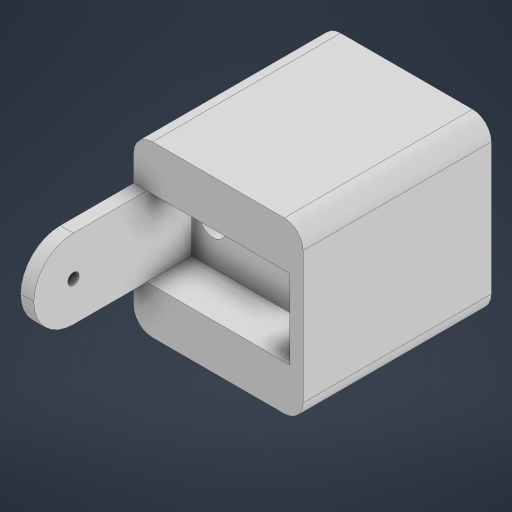
# Autodesk Inventor part: Motor holder
Saved by Autodesk Inventor 2023 (Build 270158000, 158)
## iProperties
Created: 2023-04-10
Part Number: Motor holder
Material: Generic
Document SubType Name: Modeling
Designer: vatdu
Density: 1 g/cm^3
Appearance: Default
Author: vatdu
Autodesk Inventor part; units mm, degrees
ref_plane "YZ Plane" through (0, 0, 0) normal (1, 0, 0) x (0, 1, 0)
ref_plane "XZ Plane" through (0, 0, 0) normal (0, 1, 0) x (-1, 0, 0)
ref_plane "XY Plane" through (0, 0, 0) normal (0, 0, 1) x (1, 0, 0)
sketch "Sketch1" plane through (0, 0, 0) normal (0, 0, 1) x (1, 0, 0)
  line L0 (0, 0) -> (45, 0)
  line L1 (45, 0) -> (45, 45)
  line L2 (45, 45) -> (0, 45)
  line L3 (0, 45) -> (0, 0)
  dimension "d0" = 45
  dimension "d1" = 45
  constraints: 8 end point, 2 parallel, 1 horizontal, 1 perpendicular
  measures "d0" distance of L2.end L1.end
  measures "d1" distance of L1.end L0.end
extrude "Extrusion1" add sketch "Sketch1" along normal blind 50
fillet "Fillet1" radius 5 4 edges at (45, 45, 25) (0, 45, 25) (45, 0, 25) (0, 0, 25)
sketch "Sketch2" plane through (0, 0, 0) normal (0, 0, -1) x (-1, 0, 0)
  line L0 (-45, 5) -> (-45, 40) projected
  line L1 (-45, 22.5) -> (-22.5, 22.5)
  circle A0 centre (-22.5, 22.5) radius 7.5
  point P0 (0, 0)
  dimension "d5" = 22.5
  dimension "d6" = 15
  constraints: 2 end point, 1 centre point, 1 coincident, 1 horizontal, 1 midpoint
  measures "d5" distance of L1.start L1.end
  measures "d6" diameter of A0
extrude "Extrusion2" cut sketch "Sketch2" against normal blind 20
sketch "Sketch3" plane through (0, 0, 50) normal (0, 0, 1) x (1, 0, 0)
  line L0 (0, 0) -> (3.5, 0)
  line L1 (5, 0) -> (40, 0) projected
  line L2 (3.5, 0) -> (3.5, 12)
  line L3 (3.5, 12) -> (41.5, 12)
  line L4 (41.5, 12) -> (41.5, 33)
  line L5 (41.5, 33) -> (3.5, 33)
  line L6 (3.5, 33) -> (3.5, 12)
  dimension "d11" = 3.5
  dimension "d12" = 12
  dimension "d13" = 38
  dimension "d14" = 21
  constraints: 12 end point, 2 parallel, 2 perpendicular, 1 collinear, 1 horizontal
  measures "d11" distance of L0.start L0.end
  measures "d12" distance of L0.end L2.end
  measures "d13" distance of L5.end L4.end
  measures "d14" distance of L4.end L3.end
extrude "Extrusion3" cut sketch "Sketch3" against normal blind 12
sketch "Sketch4" plane through (0, 0, 38) normal (0, 0, 1) x (1, 0, 0)
  line L0 (3.5, 12) -> (3.5, 33) projected
  line L1 (3.5, 22.5) -> (29.5, 22.5)
  line L2 (29.5, 22.5) -> (33.5, 22.5)
  line L3 (3.5, 33) -> (41.5, 33) projected
  line L4 (30.5, 33) -> (37.7775, 33)
  line L5 (37.7775, 33) -> (37.7775, 12)
  line L6 (37.7775, 12) -> (30.5, 12)
  line L7 (30.5, 12) -> (30.5, 33)
  point P0 (0, 0)
  dimension "d20" = 26
  dimension "d21" = 4
  constraints: 12 end point, 2 horizontal, 2 parallel, 2 point on line, 1 midpoint, 1 perpendicular
  measures "d20" distance of L1.start L1.end
  measures "d21" distance of L1.end L2.end
extrude "Extrusion4" cut sketch "Sketch4" against normal blind 7 contours L3 L5 L6 L7
sketch "Sketch5" plane through (0, 0, 38) normal (0, 0, 1) x (1, 0, 0)
  circle A0 centre (9.0685, 22.5) radius 3.5
  point P0 (0, 0)
  dimension "d24" = 7
  constraints: 1 centre point
  measures "d24" diameter of A0
extrude "Extrusion5" cut sketch "Sketch5" against normal blind 40
sketch "Sketch6" plane through (0, 0, 50) normal (0, 0, 1) x (1, 0, 0)
  line L0 (3.5, 33) -> (30.5, 33) projected
  line L1 (3.5, 33) -> (0, 33)
  line L2 (0, 40) -> (0, 5) projected
  line L3 (3.5, 11.9982) -> (0, 11.9982)
  line L4 (0, 33) -> (3.5, 33)
  line L5 (3.5, 33) -> (3.5, 11.9982)
  line L6 (3.5, 11.9982) -> (0, 11.9982)
  line L7 (0, 11.9982) -> (0, 33)
  point P0 (0, 0)
  constraints: 12 end point, 3 parallel, 2 horizontal, 2 point on line, 1 perpendicular
extrude "Extrusion6" add sketch "Sketch6" along normal blind 30
fillet "Fillet2" radius 10.5 2 edges at (1.75, 33, 80) (1.75, 11.9982, 80)
sketch "Sketch7" plane through (0, 5, 0) normal (-1, 0, 0) x (0, 0, 1)
  arc A0 (80, 17.5) -> (69.5, 28) centre (69.5, 17.5) ccw projected
  circle A1 centre (69.5, 17.5) radius 1.5
  point P0 (0, -5)
  dimension "d30" = 3
  constraints: 1 centre point, 1 coincident
  measures "d30" diameter of A1
extrude "Extrusion7" cut sketch "Sketch7" against normal blind 30
body "Solid1"
